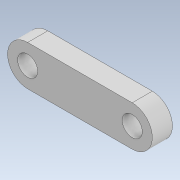
# Autodesk Inventor part: 從動件
Saved by Autodesk Inventor 2022 (Build 260153000, 153)
## iProperties
Created: 2023-05-12
Part Number: 從動件
Material: 一般
Document SubType Name: Modeling
Designer: JOU
Density: 1 g/cm^3
Appearance: 預設
Author: JOU
Autodesk Inventor part; units mm, degrees
ref_plane "YZ Plane" through (0, 0, 0) normal (1, 0, 0) x (0, 1, 0)
ref_plane "XZ Plane" through (0, 0, 0) normal (0, 1, 0) x (-1, 0, 0)
ref_plane "XY Plane" through (0, 0, 0) normal (0, 0, 1) x (1, 0, 0)
sketch "草圖1" plane through (0, 0, 0) normal (0, 0, 1) x (1, 0, 0)
  circle A0 centre (0, 0) radius 5
  line L0 (0, 0) -> (52, 0) construction
  line L1 (0, -10) -> (52, -10)
  line L2 (52, 10) -> (0, 10)
  arc A1 (0, 10) -> (0, -10) centre (0, 0) ccw
  arc A2 (52, -10) -> (52, 10) centre (52, 0) ccw
  circle A3 centre (52, 0) radius 5
  point P0 (26, 0)
  dimension "d0" = 10
  dimension "d1" = 20
  dimension "d2" = 52
  dimension "d3" = 10
  constraints: 8 end point, 4 centre point, 4 point on circle, 4 tangent, 2 coincident, 1 horizontal, 1 midpoint, 1 parallel
  measures "d0" diameter of A0
  measures "d1" distance between parallel lines of L1 L2
  measures "d2" distance of L0.start L0.end
  measures "d3" diameter of A3
extrude "擠出1" add sketch "草圖1" along normal blind 10
